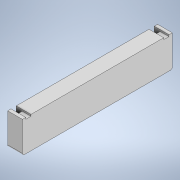
# Autodesk Inventor part: Front
Saved by Autodesk Inventor 2022 (Build 260153000, 153)
## iProperties
Created: 2022-06-23
Part Number: Front
Material: Generic
Document SubType Name: Modeling
Designer: abdoo
Density: 1 g/cm^3
Appearance: Default
Author: abdoo
Autodesk Inventor part; units mm, degrees
ref_plane "YZ Plane" through (0, 0, 0) normal (1, 0, 0) x (0, 1, 0)
ref_plane "XZ Plane" through (0, 0, 0) normal (0, 1, 0) x (-1, 0, 0)
ref_plane "XY Plane" through (0, 0, 0) normal (0, 0, 1) x (1, 0, 0)
sketch "Sketch1" plane through (0, 0, 0) normal (1, 0, 0) x (0, 1, 0)
  line L0 (0, 0) -> (3, 0)
  line L1 (3, 0) -> (3, -87.28)
  line L2 (3, -87.28) -> (0, -87.28)
  line L3 (0, -87.28) -> (0, 0)
  line L4 (3.125, -87.405) -> (3.125, 0.125)
  line L5 (3.125, 0.125) -> (-0.125, 0.125)
  line L6 (-0.125, 0.125) -> (-0.125, -87.405)
  line L7 (-0.125, -87.405) -> (3.125, -87.405)
  line L8 (5.125, 2.125) -> (5.125, -89.405)
  line L9 (5.125, -89.405) -> (-2.125, -89.405)
  line L10 (-2.125, -89.405) -> (-2.125, 2.125)
  line L11 (-2.125, 2.125) -> (5.125, 2.125)
  line L12 (3, -87.28) -> (15, -87.28)
  line L13 (15, -87.28) -> (15, -84.28)
  line L14 (15, -84.28) -> (3, -84.28)
  line L15 (3, -84.28) -> (3, -87.28)
  line L16 (3, 0) -> (15, 0)
  line L17 (15, 0) -> (15, -3)
  line L18 (15, -3) -> (3, -3)
  line L19 (3, -3) -> (3, 0)
  line L20 (15.1, 0.1) -> (2.9, 0.1)
  line L21 (2.9, 0.1) -> (2.9, -3.1)
  line L22 (2.9, -3.1) -> (15.1, -3.1)
  line L23 (15.1, -3.1) -> (15.1, 0.1)
  line L24 (15.1, -87.38) -> (2.9, -87.38)
  line L25 (2.9, -87.38) -> (2.9, -84.18)
  line L26 (2.9, -84.18) -> (15.1, -84.18)
  line L27 (15.1, -84.18) -> (15.1, -87.38)
  line L28 (0.875, -89.405) -> (17.125, -89.405)
  line L29 (17.125, -89.405) -> (17.125, -82.155)
  line L30 (17.125, -82.155) -> (0.875, -82.155)
  line L31 (0.875, -82.155) -> (0.875, -89.405)
  line L32 (17.125, 2.125) -> (0.875, 2.125)
  line L33 (0.875, 2.125) -> (0.875, -5.125)
  line L34 (0.875, -5.125) -> (17.125, -5.125)
  line L35 (17.125, -5.125) -> (17.125, 2.125)
  line L36 (15.1, 0.1) -> (17.125, 0.1)
  line L37 (15.1, -3.1) -> (17.125, -3.1)
  line L38 (15.1, -87.38) -> (17.125, -87.38)
  line L39 (15.1, -84.18) -> (17.125, -84.18)
  point P0 (5.125, -82.155)
  point P1 (5.125, -5.125)
  point P2 (3.125, -84.18)
  point P3 (3.125, -87.38)
  point P4 (3.125, 0.1)
  point P5 (3.125, -3.1)
  dimension "d0" = 87.28
  dimension "d1" = 3
  dimension "d2" = 0.125
  dimension "d3" = 2
  dimension "d4" = 12
  dimension "d5" = 3
  dimension "d6" = 12
  dimension "d7" = 3
  dimension "d8" = 0.1
  dimension "d9" = 0.1
  dimension "d10" = 0
  dimension "d11" = 0
  constraints: 80 end point, 18 parallel, 12 perpendicular, 4 horizontal, 4 point on line, 18 other
  measures "d0" distance of L0.end L1.end
  measures "d1" distance of L1.end L2.end
  measures "d2" distance between parallel lines of L1 L4
  measures "d3" distance between parallel lines of L4 L8
  measures "d4" distance of L1.end L12.end
  measures "d5" distance of L12.end L13.end
  measures "d6" distance of L17.end L18.end
  measures "d7" distance of L16.end L17.end
  measures "d8" distance between parallel lines of L16 L20
  measures "d9" distance between parallel lines of L12 L24
  measures "d10" distance between parallel lines of L11 L32
  measures "d11" distance between parallel lines of L9 L28
extrude "Extrusion1" add sketch "Sketch1" along normal blind 6.5 contours L33 L11 L8 L20 L4 L5 | L5 L6 L7 L31 L9 L10 L11 L33 | L7 L4 L24 L8 L9 L31 | L32 L35 L36 L20 L8 | L34 L8 L30 L4 | L4 L22 L8 L34 | L30 L8 L26 L4 | L8 L22 L37 L35 L34 | L8 L24 L38 L29 L28 | L30 L29 L39 L26 L8
sketch "Sketch2" plane through (6.5, 0, 0) normal (1, 0, 0) x (0, 0, -1)
  line L0 (3.1, 16.125) -> (-0.1, 16.125)
  line L1 (-0.1, 16.125) -> (-0.1, 3.325)
  line L2 (-0.1, 3.325) -> (3.1, 3.325)
  line L3 (3.1, 3.325) -> (3.1, 16.125)
  line L4 (3.1, 3.125) -> (84.18, 3.125) projected
  line L5 (5.125, 17.125) -> (3.1, 17.125) projected
  line L6 (-0.1, 3.125) -> (-0.1, 17.125) projected
  line L7 (3.1, 17.125) -> (3.1, 3.125) projected
  line L8 (84.18, 3.325) -> (87.38, 3.325)
  line L9 (87.38, 3.325) -> (87.38, 16.125)
  line L10 (87.38, 16.125) -> (84.18, 16.125)
  line L11 (84.18, 16.125) -> (84.18, 3.325)
  line L12 (89.405, 17.125) -> (87.38, 17.125) projected
  line L13 (87.38, 17.125) -> (87.38, 3.125) projected
  line L14 (84.18, 3.125) -> (84.18, 17.125) projected
  line L15 (28.765, -0.125) -> (58.515, -0.125)
  line L16 (58.515, -0.125) -> (58.515, 3.125)
  line L17 (58.515, 3.125) -> (28.765, 3.125)
  line L18 (28.765, 3.125) -> (28.765, -0.125)
  line L19 (87.405, -0.125) -> (-0.125, -0.125) projected
  line L20 (-0.125, -0.125) -> (-0.125, 3.125) projected
  point P0 (0, 0)
  dimension "d14" = 0.2
  dimension "d15" = 1
  dimension "d16" = 0
  dimension "d17" = 0
  dimension "d18" = 0.2
  dimension "d19" = 1
  dimension "d20" = 0
  dimension "d21" = 0
  dimension "d22" = 29.75
  dimension "d23" = 0
  dimension "d24" = 0
  dimension "d25" = 28.89
  constraints: 24 end point, 6 parallel, 3 horizontal, 3 perpendicular
  measures "d14" distance from line of L4 L2.end
  measures "d15" distance between parallel lines of L5 L0
  measures "d16" distance between parallel lines of L6 L1
  measures "d17" distance between parallel lines of L7 L3
  measures "d18" distance between parallel lines of L4 L8
  measures "d19" distance from line of L12 L9.end
  measures "d20" distance between parallel lines of L13 L9
  measures "d21" distance between parallel lines of L14 L11
  measures "d22" distance of L16.end L17.end
  measures "d23" distance between parallel lines of L4 L17
  measures "d24" distance between parallel lines of L19 L15
  measures "d25" distance between parallel lines of L20 L18
extrude "Extrusion2" add sketch "Sketch2" against normal blind 2.85
sketch "Sketch3" plane through (6.5, 0, 0) normal (1, 0, 0) x (0, 0, -1)
  line L0 (84.18, 16.125) -> (84.18, 17.125) projected
  line L1 (84.18, 17.125) -> (82.155, 17.125) projected
  line L2 (82.155, 17.125) -> (82.155, 5.125) projected
  line L3 (82.155, 5.125) -> (5.125, 5.125) projected
  line L4 (5.125, 5.125) -> (5.125, 17.125) projected
  line L5 (5.125, 17.125) -> (3.1, 17.125) projected
  line L6 (3.1, 17.125) -> (3.1, 16.125) projected
  line L7 (3.1, 16.125) -> (-0.1, 16.125) projected
  line L8 (-0.1, 16.125) -> (-0.1, 17.125) projected
  line L9 (-0.1, 17.125) -> (-2.125, 17.125) projected
  line L10 (-2.125, 17.125) -> (-2.125, -2.125) projected
  line L11 (-2.125, -2.125) -> (89.405, -2.125) projected
  line L12 (89.405, -2.125) -> (89.405, 17.125) projected
  line L13 (89.405, 17.125) -> (87.38, 17.125) projected
  line L14 (87.38, 17.125) -> (87.38, 16.125) projected
  line L15 (87.38, 16.125) -> (84.18, 16.125) projected
  line L16 (84.18, 3.325) -> (87.38, 3.325) projected
  line L17 (87.38, 3.325) -> (87.38, 3.125) projected
  line L18 (87.38, 3.125) -> (87.405, 3.125) projected
  line L19 (87.405, 3.125) -> (87.405, -0.125) projected
  line L20 (87.405, -0.125) -> (58.515, -0.125) projected
  line L21 (58.515, -0.125) -> (58.515, 3.125) projected
  line L22 (58.515, 3.125) -> (84.18, 3.125) projected
  line L23 (84.18, 3.125) -> (84.18, 3.325) projected
  line L24 (28.765, 3.125) -> (28.765, -0.125) projected
  line L25 (28.765, -0.125) -> (-0.125, -0.125) projected
  line L26 (-0.125, -0.125) -> (-0.125, 3.125) projected
  line L27 (-0.125, 3.125) -> (-0.1, 3.125) projected
  line L28 (-0.1, 3.125) -> (-0.1, 3.325) projected
  line L29 (-0.1, 3.325) -> (3.1, 3.325) projected
  line L30 (3.1, 3.325) -> (3.1, 3.125) projected
  line L31 (3.1, 3.125) -> (28.765, 3.125) projected
  point P0 (0, 0)
extrude "Extrusion4" add sketch "Sketch3" along normal blind 2.5 contours L15 L14 L13 L12 L11 L10 L9 L8 L7 L6 L5 L4 L3 L2 L1 L0 | L16 L17 L18 L19 L20 L21 L22 L23 | L24 L25 L26 L27 L28 L29 L30 L31
sketch "Sketch4" plane through (0, 0, 0) normal (-1, 0, 0) x (0, 0, 1)
  line L0 (-5.125, 5.125) -> (-5.125, 17.125) projected
  line L1 (-82.155, 17.125) -> (-82.155, 5.125) projected
  line L2 (-5.125, 5.125) -> (-82.155, 5.125)
  line L3 (-82.155, 5.125) -> (-82.155, 17.125)
  line L4 (-82.155, 17.125) -> (-5.125, 17.125)
  line L5 (-5.125, 17.125) -> (-5.125, 5.125)
  point P0 (0, 0)
  constraints: 8 end point, 2 parallel, 1 horizontal, 1 perpendicular
extrude "Extrusion5" add sketch "Sketch4" against normal up to surface (9 mm away)
fillet "Fillet1" radius 1.25 2 edges at (4.5, -2.125, 2.125) (4.5, -2.125, -89.405)
body "Solid1"
